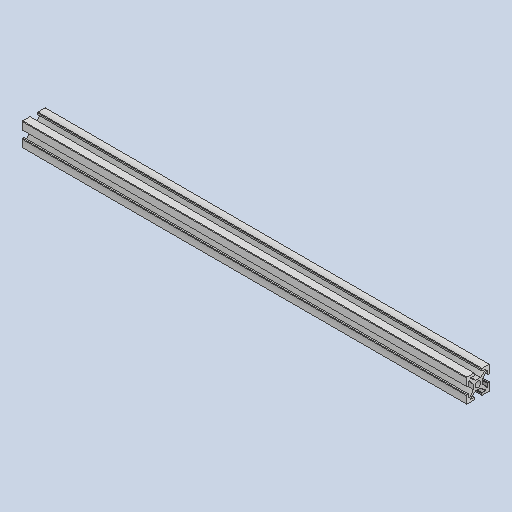
# Autodesk Inventor part: profile190
Saved by Autodesk Inventor 2023 (Build 270158000, 158)
## iProperties
Created: 2023-11-05
Part Number: profile190
Material: Générique
Document SubType Name: Modeling
Designer: eleves
Density: 1 g/cm^3
Appearance: Par défaut
Author: eleves
Autodesk Inventor part; units mm, degrees
ref_plane "YZ Plane" through (0, 0, 0) normal (1, 0, 0) x (0, 1, 0)
ref_plane "XZ Plane" through (0, 0, 0) normal (0, 1, 0) x (-1, 0, 0)
ref_plane "XY Plane" through (0, 0, 0) normal (0, 0, 1) x (1, 0, 0)
sketch "Esquisse1" plane through (0, 0, 0) normal (1, 0, 0) x (0, 1, 0)
  line L0 (-5, -5) -> (5, 5) construction
  line L1 (5, -5) -> (-5, 5) construction
  circle A0 centre (0, 0) radius 1.25
  line L2 (2, 1) -> (2, -1)
  line L3 (-1, 2) -> (1, 2)
  line L4 (-2, -1) -> (-2, 1)
  line L5 (1, -2) -> (-1, -2)
  line L6 (4.8, -5) -> (1.7, -5)
  line L7 (5, -4.8) -> (5, -1.7)
  line L8 (1.5, -4.8) -> (1.5, -4.2)
  line L9 (12.6837, 0) -> (-8.9006, 0) construction
  line L10 (1.5, -4) -> (4, -4) construction
  line L11 (4, -4) -> (4, -1.5) construction
  line L12 (4, -1.5) -> (5, -1.5) construction
  line L13 (5, -5) -> (2, -1) construction
  line L14 (2, -1) -> (4, -3.6667) construction
  line L15 (2, -1) -> (4, -3.6667) construction
  line L16 (4, -3.0667) -> (4, -1.7)
  line L17 (4.8, -1.5) -> (4.2, -1.5)
  line L18 (1, -2) -> (5, -5) construction
  line L19 (1.7, -4) -> (3.0667, -4)
  line L20 (3.1867, -3.64) -> (1, -2)
  line L21 (2, -1) -> (3.64, -3.1867)
  arc A1 (5, -1.7) -> (4.8, -1.5) centre (4.8, -1.7) ccw
  arc A2 (4.2, -1.5) -> (4, -1.7) centre (4.2, -1.7) ccw
  arc A3 (4.8, -5) -> (5, -4.8) centre (4.8, -4.8) ccw
  arc A4 (1.5, -4.8) -> (1.7, -5) centre (1.7, -4.8) ccw
  arc A5 (1.7, -4) -> (1.5, -4.2) centre (1.7, -4.2) ccw
  arc A6 (3.0667, -4) -> (3.1867, -3.64) centre (3.0667, -3.8) ccw
  arc A7 (3.64, -3.1867) -> (4, -3.0667) centre (3.8, -3.0667) ccw
  arc A8 (3.1867, 3.64) -> (3.0667, 4) centre (3.0667, 3.8) ccw
  line L22 (1.5, 4.8) -> (1.5, 4.2)
  line L23 (1.5, 4) -> (1.5, 5) construction
  arc A9 (4, 3.0667) -> (3.64, 3.1867) centre (3.8, 3.0667) ccw
  line L24 (3.0667, 4) -> (1.7, 4)
  arc A10 (1.5, 4.2) -> (1.7, 4) centre (1.7, 4.2) ccw
  line L25 (4, 1.7) -> (4, 3.0667)
  line L26 (4, 4) -> (1.5, 4) construction
  line L27 (1, 2) -> (3.1867, 3.64)
  line L28 (4.8, 1.5) -> (4.2, 1.5)
  line L29 (1, 2) -> (3.6667, 4) construction
  line L30 (1, 2) -> (3.6667, 4) construction
  line L31 (4.8, 5) -> (1.7, 5)
  line L32 (3.64, 3.1867) -> (2, 1)
  line L33 (5, 4.8) -> (5, 1.7)
  line L34 (5, 5) -> (1, 2) construction
  line L35 (2, 1) -> (5, 5) construction
  line L36 (4, 1.5) -> (4, 4) construction
  circle A11 centre (0, 0) radius 1.25
  line L37 (-1, 2) -> (1, 2)
  line L38 (-2, -1) -> (-2, 1)
  line L39 (1, -2) -> (-1, -2)
  line L40 (2, 1) -> (2, -1)
  arc A12 (1.7, 5) -> (1.5, 4.8) centre (1.7, 4.8) ccw
  arc A13 (5, 4.8) -> (4.8, 5) centre (4.8, 4.8) ccw
  arc A14 (4, 1.7) -> (4.2, 1.5) centre (4.2, 1.7) ccw
  arc A15 (4.8, 1.5) -> (5, 1.7) centre (4.8, 1.7) ccw
  arc A16 (-3.64, 3.1867) -> (-4, 3.0667) centre (-3.8, 3.0667) ccw
  line L41 (-4.8, 1.5) -> (-4.2, 1.5)
  line L42 (-4, 1.5) -> (-5, 1.5) construction
  arc A17 (-3.0667, 4) -> (-3.1867, 3.64) centre (-3.0667, 3.8) ccw
  line L43 (-4, 3.0667) -> (-4, 1.7)
  arc A18 (-4.2, 1.5) -> (-4, 1.7) centre (-4.2, 1.7) ccw
  line L44 (-1.7, 4) -> (-3.0667, 4)
  line L45 (-4, 4) -> (-4, 1.5) construction
  line L46 (-2, 1) -> (-3.64, 3.1867)
  line L47 (-1.5, 4.8) -> (-1.5, 4.2)
  line L48 (-2, 1) -> (-4, 3.6667) construction
  line L49 (-2, 1) -> (-4, 3.6667) construction
  line L50 (-5, 4.8) -> (-5, 1.7)
  line L51 (-3.1867, 3.64) -> (-1, 2)
  line L52 (-4.8, 5) -> (-1.7, 5)
  line L53 (-5, 5) -> (-2, 1) construction
  line L54 (-1, 2) -> (-5, 5) construction
  line L55 (-1.5, 4) -> (-4, 4) construction
  circle A19 centre (0, 0) radius 1.25
  line L56 (-2, -1) -> (-2, 1)
  line L57 (1, -2) -> (-1, -2)
  line L58 (2, 1) -> (2, -1)
  line L59 (-1, 2) -> (1, 2)
  arc A20 (-5, 1.7) -> (-4.8, 1.5) centre (-4.8, 1.7) ccw
  arc A21 (-4.8, 5) -> (-5, 4.8) centre (-4.8, 4.8) ccw
  arc A22 (-1.7, 4) -> (-1.5, 4.2) centre (-1.7, 4.2) ccw
  arc A23 (-1.5, 4.8) -> (-1.7, 5) centre (-1.7, 4.8) ccw
  arc A24 (-3.1867, -3.64) -> (-3.0667, -4) centre (-3.0667, -3.8) ccw
  line L60 (-1.5, -4.8) -> (-1.5, -4.2)
  line L61 (-1.5, -4) -> (-1.5, -5) construction
  arc A25 (-4, -3.0667) -> (-3.64, -3.1867) centre (-3.8, -3.0667) ccw
  line L62 (-3.0667, -4) -> (-1.7, -4)
  arc A26 (-1.5, -4.2) -> (-1.7, -4) centre (-1.7, -4.2) ccw
  line L63 (-4, -1.7) -> (-4, -3.0667)
  line L64 (-4, -4) -> (-1.5, -4) construction
  line L65 (-1, -2) -> (-3.1867, -3.64)
  line L66 (-4.8, -1.5) -> (-4.2, -1.5)
  line L67 (-1, -2) -> (-3.6667, -4) construction
  line L68 (-1, -2) -> (-3.6667, -4) construction
  line L69 (-4.8, -5) -> (-1.7, -5)
  line L70 (-3.64, -3.1867) -> (-2, -1)
  line L71 (-5, -4.8) -> (-5, -1.7)
  line L72 (-5, -5) -> (-1, -2) construction
  line L73 (-2, -1) -> (-5, -5) construction
  line L74 (-4, -1.5) -> (-4, -4) construction
  circle A27 centre (0, 0) radius 1.25
  line L75 (1, -2) -> (-1, -2)
  line L76 (2, 1) -> (2, -1)
  line L77 (-1, 2) -> (1, 2)
  line L78 (-2, -1) -> (-2, 1)
  arc A28 (-1.7, -5) -> (-1.5, -4.8) centre (-1.7, -4.8) ccw
  arc A29 (-5, -4.8) -> (-4.8, -5) centre (-4.8, -4.8) ccw
  arc A30 (-4, -1.7) -> (-4.2, -1.5) centre (-4.2, -1.7) ccw
  arc A31 (-4.8, -1.5) -> (-5, -1.7) centre (-4.8, -1.7) ccw
  point P0 (2, 0)
  point P1 (0, 2)
  point P2 (-2, 0)
  point P3 (0, -2)
  point P4 (1.5, -5)
  point P5 (3.6667, -4)
  point P6 (4, 3.6667)
  point P7 (5, 1.5)
  point P8 (0, 2)
  point P9 (-2, 0)
  point P10 (0, -2)
  point P11 (2, 0)
  point P12 (-3.6667, 4)
  point P13 (-1.5, 5)
  point P14 (-2, 0)
  point P15 (0, -2)
  point P16 (2, 0)
  point P17 (0, 2)
  point P18 (-4, -3.6667)
  point P19 (-5, -1.5)
  point P20 (0, -2)
  point P21 (2, 0)
  point P22 (0, 2)
  point P23 (-2, 0)
  dimension "d0" = 10
  dimension "d1" = 10
  dimension "d19" = 2.5
  dimension "d30" = 2
  dimension "d36" = 360
  dimension "d39" = 3.5
  dimension "d40" = 3.5
  dimension "d41" = 1
  dimension "d50" = 0.2
  dimension "d60" = 0.2
  dimension "d61" = 0.2
  dimension "d62" = 0.2
  dimension "d63" = 0.2
  dimension "d64" = 0.2
  dimension "d73" = 0.2
  dimension "d80" = 360
  constraints: 158 end point, 73 point on line, 56 point on circle, 32 centre point, 14 tangent, 6 coincident, 5 perpendicular, 3 midpoint, 2 collinear, 2 horizontal, 2 vertical, 1 parallel, 296 other
  measures "d0" distance of L1.start L0.end
  measures "d1" distance of L0.end L1.end
  measures "d19" diameter of A0
  measures "d30" distance of L2.start L2.end
  measures "d39" distance of L1.start point (1.5, -5)
  measures "d40" distance of L1.start L12.end
  measures "d41" distance of point (1.5, -5) L10.start
  measures "d50" radius of A1
  measures "d60" radius of A2
  measures "d61" radius of A3
  measures "d62" radius of A4
  measures "d63" radius of A5
  measures "d64" radius of A6
  measures "d73" radius of A7
extrude "Extrusion1" add sketch "Esquisse1" along normal blind 190
